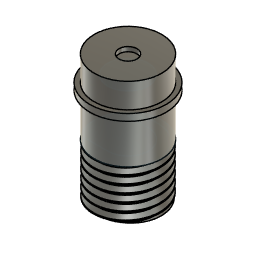
Initial axle design v1 (Autodesk Fusion 360 design; units mm, degrees)
Autodesk Fusion 360 part; units mm, degrees
sketch "Sketch1" plane through (0, 0, 0) normal (0, 0, 1) x (1, 0, 0)
  circle A0 centre (0, 0) radius 15
  dimension "d1" = 30
  constraint coincident A0.centre origin
  measures "d1" diameter of A0
extrude "Extrude1" add sketch "Sketch1" along normal blind 23
sketch "Sketch2" plane through (0, 0, 23) normal (0, 0, 1) x (-1, 0, 0)
  circle A0 centre (0, 0) radius 15
  circle A1 centre (0, 0) radius 15
  dimension "d4" = 30
  constraint concentric A0 A1
  measures "d4" diameter of A1
sketch "Sketch3" plane through (0, 0, 0) normal (0, 0, -1) x (1, 0, 0)
  circle A0 centre (0, 0) radius 15
  circle A1 centre (0, 0) radius 9
  line L0 (0, 9) -> (-15, 9)
  line L1 (-15, 9) -> (-15, -9)
  line L2 (-15, -9) -> (0, -9)
  line L3 (0, -9) -> (0, 9)
  dimension "d5" = 18
  dimension "d21" = 18
  constraint concentric A0 A1
  constraint horizontal L0
  constraint vertical L1
  constraint horizontal L2
  constraint vertical L3
  constraint coincident A1 L0.start
  measures "d5" diameter of A1
  measures "d21" distance of L0.start L2.end
extrude "Extrude2" cut sketch "Sketch3" against normal blind 23 contours A0 A1 L0 L2 | A1 L3 | A1 L3 picked at (-12.9503, -0.8659)
thread "Thread1" "ISO Metric profile 30.0 M30x3.5 6g" major diameter 29.7345 minor diameter 25.732 pitch 3.5 angle 60 modelled right hand crest width 0.4992 on face at (-11.5449, -9.5768, 15.3333) crest through (14.8673, 0, -0.875)
sketch "Sketch4" plane through (0, 0, 23) normal (0, 0, 1) x (-1, 0, 0)
extrude "Extrude3" add sketch "Sketch2" along normal blind 19
sketch "Sketch5" plane through (0, 0, 42) normal (0, 0, 1) x (-1, 0, 0)
  circle A0 centre (0, 0) radius 15
  circle A1 centre (0, 0) radius 17
  dimension "d12" = 34
  constraint concentric A0 A1
  measures "d12" diameter of A1
extrude "Extrude4" add sketch "Sketch5" along normal blind 3 contours A0 | A1
sketch "Sketch6" plane through (0, 0, 45) normal (0, 0, 1) x (-1, 0, 0)
  circle A0 centre (0, 0) radius 17
  circle A1 centre (0, 0) radius 15
  dimension "d15" = 30
  constraint coincident A0.centre A1.centre
  measures "d15" diameter of A1
extrude "Extrude5" add sketch "Sketch6" along normal blind 11 contours A1
sketch "Sketch7" plane through (0, 0, 56) normal (0, 0, 1) x (-1, 0, 0)
  circle A0 centre (0, 0) radius 15
  circle A1 centre (0, 0) radius 4
  dimension "d18" = 8
  constraint concentric A0 A1
  measures "d18" diameter of A1
extrude "Extrude6" cut sketch "Sketch7" against normal blind 2 contours A1
sketch "Sketch8" plane through (0, 0, 23) normal (0, 0, -1) x (1, 0, 0)
  circle A0 centre (0, 0) radius 15
  spline S0 degree 3 poles (-10.7542, 9) (-10.3236, 9.5929) (-9.8461, 10.1524) (-8.1054, 11.8955) (-6.6715, 12.8838) (-3.486, 14.3257) (-1.7548, 14.754) (0.0111, 14.8672) knots 0.324156 0.324156 0.324156 0.324156 0.544902 0.544902 1.062753 1.062753 1.592832 1.592832 1.592832 1.592832
  arc A1 (11.6168, 9.2782) -> (0.0111, 14.8672) centre (0, 0) ccw
  spline S1 degree 3 poles (11.6168, 9.2782) (12.7086, 7.7131) (13.4881, 5.9523) (14.309, 2.276) (14.3603, 0.4003) (13.7403, -3.2161) (13.0932, -4.9248) (11.1983, -7.9522) (9.9845, -9.2513) (7.6103, -10.9538) (6.5828, -11.504) (4.4303, -12.3116) (3.3166, -12.5706) (2.1834, -12.6794) knots 0 0 0 0 0.572495 0.572495 1.130652 1.130652 1.674465 1.674465 2.203926 2.203926 2.552907 2.552907 2.895334 2.895334 2.895334 2.895334
  arc A2 (-9.1942, -9) -> (2.1834, -12.6794) centre (0, 0) ccw
  line L0 (-9.1942, -9) -> (0, -9)
  arc A3 (0, -9) -> (0, 9) centre (0, 0) ccw
  line L1 (0, 9) -> (-10.7542, 9)
sketch "Sketch9" plane through (0, 0, 23) normal (0, 0, -1) x (1, 0, 0)
  circle A0 centre (0, 0) radius 9
  dimension "d22" = 18
  constraint coincident A0.centre origin
  measures "d22" diameter of A0
extrude "Extrude7" cut sketch "Sketch9" against normal blind 25
sketch "Sketch10" plane through (0, 0, 48) normal (0, 0, -1) x (1, 0, 0)
  circle A0 centre (0, 0) radius 9
